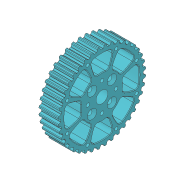
# Autodesk Inventor part: TIMING_BELT_P40
Saved by Autodesk Inventor 2019.4 (Build 234330000, 330)
## iProperties
Created: 2019-11-09
Part Number: TIMING_BELT_P40
Material: 一般
Document SubType Name: Modeling
Designer: y6tada
Density: 1 g/cm^3
Appearance: くすんだ青
Author: y6tada
Autodesk Inventor part; units mm, degrees
ref_plane "YZ Plane" through (0, 0, 0) normal (1, 0, 0) x (0, 1, 0)
ref_plane "XZ Plane" through (0, 0, 0) normal (0, 1, 0) x (-1, 0, 0)
ref_plane "XY Plane" through (0, 0, 0) normal (0, 0, 1) x (1, 0, 0)
sketch "スケッチ1" plane through (0, 0, 0) normal (1, 0, 0) x (0, 1, 0)
  arc A0 (0.9801, -18.6943) -> (0, -18.72) centre (0, 0) ccw construction
  line L0 (0, 0) -> (0, -15.5638) construction
  line L1 (0.975, -18.974) -> (-0.975, -18.974) construction
  arc A1 (0.9801, -18.6943) -> (0.4479, -17.6043) centre (-0.975, -18.974) ccw
  arc A2 (-0.4479, -17.6043) -> (0.4479, -17.6043) centre (0, 0) ccw
  arc A3 (-0.4479, -17.6043) -> (-0.9801, -18.6943) centre (0.975, -18.974) ccw
  circle A4 centre (0, 0) radius 14.32 construction
  line L2 (0, -18.72) -> (0.975, -18.72) construction
  circle A5 centre (0, 0) radius 19.1 construction
  line L3 (1.4688, -18.6623) -> (0, 0)
  line L4 (0, 0) -> (-1.4688, -18.6623)
  arc A6 (-1.4688, -18.6623) -> (-0.9801, -18.6943) centre (0, 0) ccw
  arc A7 (0.9801, -18.6943) -> (1.4688, -18.6623) centre (0, 0) ccw
  dimension "d2" = 1.95
  dimension "d3" = 1.975
  dimension "d4" = 1.11
  dimension "d8" = 0.254
  dimension "d10" = 37.44
  dimension "d11" = 38.2
  dimension "d12" = 9
  constraints: 14 point on circle, 10 end point, 8 centre point, 4 symmetric about line, 3 coincident, 1 concentric, 1 horizontal, 1 perpendicular, 1 point on line, 1 tangent, 1 vertical, 1 other
  measures "d2" distance of L1.start L1.end
  measures "d3" radius of A1
  measures "d4" radial gap between concentric circles of A0 A2
  measures "d8" distance between parallel lines of L1 L2
  measures "d10" diameter of A0
  measures "d11" diameter of A5
  measures "d12" angle of L4 L3
extrude "押し出し1" add sketch "スケッチ1" along normal blind 8.2
fillet "フィレット1" radius 0.15 2 edges at (4.1, 0.4479, -17.6043) (4.1, -0.4479, -17.6043)
fillet "フィレット2" radius 0.28 2 edges at (4.1, 0.9801, -18.6943) (4.1, -0.9801, -18.6943)
pattern_circular "円形状パターン1" count 40 over 360 about axis through (-10, 0, 0) along (1, 0, 0)
sketch "スケッチ9" plane through (0, 0, 0) normal (-1, 0, 0) x (0, 0, 1)
  circle A0 centre (0, 0) radius 14
  dimension "d79" = 28
  constraints: 1 centre point, 1 coincident
  measures "d79" diameter of A0
extrude "押し出し6" add sketch "スケッチ9" along normal blind 1
sketch "スケッチ3" plane through (-1, 0, 0) normal (-1, 0, 0) x (0, 0, 1)
  circle A0 centre (0, 0) radius 7.5
  dimension "d27" = 15
  constraints: 1 centre point, 1 coincident
  measures "d27" diameter of A0
extrude "押し出し2" add sketch "スケッチ3" along normal blind 1
sketch "スケッチ2" plane through (8.2, 0, 0) normal (1, 0, 0) x (0, 0, -1)
  point P0 (0, 0)
  point P1 (0, 0)
  constraints: 1 coincident
hole "穴1" at (8.2, 0, 0) direction (-1, 0, 0) diameter 5 end through all
sketch "スケッチ4" plane through (-2, 0, 0) normal (-1, 0, 0) x (0, 0, 1)
  circle A0 centre (0, 0) radius 6 construction
  line L0 (0, 0) -> (6, 0) construction
  point P0 (0, 6)
  point P1 (-6, 0)
  point P2 (0, -6)
  dimension "d30" = 12
  dimension "d33" = 360
  constraints: 2 end point, 1 coincident, 1 horizontal, 1 horizontal alignment, 7 other
hole "穴2" at (-2, 0, 6) at (-2, 6, 0) at (-2, 0, -6) at (-2, -6, 0) direction (1, 0, 0) diameter 1.5 end through all both
sketch "スケッチ5" plane through (8.2, 0, 0) normal (-1, 0, 0) x (0, 0, 1)
  circle A0 centre (0, 0) radius 6 construction
  line L0 (0, 0) -> (4.2426, 4.2426) construction
  line L1 (0, 0) -> (9.6781, 0) construction
  point P0 (-4.2426, 4.2426)
  point P1 (-4.2426, -4.2426)
  point P2 (4.2426, -4.2426)
  dimension "d43" = 12
  dimension "d42" = 45
  dimension "d46" = 360
  constraints: 4 end point, 2 coincident, 1 horizontal, 8 other
  measures "d42" angle of L1 L0
hole "穴3" at (8.2, 4.2426, 4.2426) at (8.2, 4.2426, -4.2426) at (8.2, -4.2426, -4.2426) at (8.2, -4.2426, 4.2426) direction (-1, 0, 0) diameter 2 end through all countersink diameter 4 countersink angle 90
sketch "スケッチ6" plane through (-1, 0, 0) normal (-1, 0, 0) x (0, 0, 1)
  circle A0 centre (0, 0) radius 8.4
  circle A1 centre (0, 0) radius 10.2
  dimension "d55" = 20.4
  dimension "d56" = 16.8
  constraints: 2 centre point, 2 coincident
  measures "d55" diameter of A1
  measures "d56" diameter of A0
extrude "押し出し3" cut sketch "スケッチ6" against normal blind 0.2
sketch "スケッチ7" plane through (-1, 0, 0) normal (-1, 0, 0) x (0, 0, 1)
  circle A0 centre (0, 0) radius 12 construction
  circle A1 centre (0, 0) radius 11.45
  circle A2 centre (0, 0) radius 12.55
  dimension "d59" = 24
  dimension "d60" = 0.55
  dimension "d61" = 0.55
  constraints: 3 centre point, 3 coincident
  measures "d59" diameter of A0
  measures "d60" radial gap between concentric circles of A0 A1
  measures "d61" radial gap between concentric circles of A2 A0
extrude "押し出し4" cut sketch "スケッチ7" against normal blind 0.5
sketch "スケッチ8" plane through (8.2, 0, 0) normal (1, 0, 0) x (0, 0, -1)
  circle A0 centre (0, 0) radius 9 construction
  circle A1 centre (0, 0) radius 16 construction
  line L0 (0, 0) -> (14.7821, 6.1229) construction
  line L1 (0, 0) -> (14.7821, -6.1229) construction
  line L2 (0, 0) -> (22.4689, 0) construction
  arc A2 (13.8872, 4.447) -> (9.7713, 3.1815) centre (18.5109, -17.9179) ccw
  arc A3 (8.8674, -1.5391) -> (8.8674, 1.5391) centre (0, 0) ccw
  arc A4 (15.6589, -3.2861) -> (15.6589, 3.2861) centre (0, 0) ccw
  arc A5 (9.7713, 3.1815) -> (8.8674, 1.5391) centre (10.3453, 1.7957) ccw
  arc A6 (15.6589, 3.2861) -> (13.8872, 4.447) centre (14.1909, 2.978) ccw
  arc A7 (9.7713, -3.1815) -> (13.8872, -4.447) centre (18.5109, 17.9179) ccw
  arc A8 (8.8674, -1.5391) -> (9.7713, -3.1815) centre (10.3453, -1.7957) ccw
  arc A9 (13.8872, -4.447) -> (15.6589, -3.2861) centre (14.1909, -2.978) ccw
  line L3 (0.6834, -0.5828) -> (15.4655, 5.5401) construction
  circle A10 centre (14.7821, 6.1229) radius 1.7 construction
  dimension "d64" = 18
  dimension "d65" = 32
  dimension "d66" = 45
  dimension "d67" = 1.5
  dimension "d69" = 1.6
  dimension "d83" = 3.4
  constraints: 18 point on circle, 11 centre point, 10 tangent, 8 end point, 5 coincident, 5 equal radius, 2 concentric, 2 symmetric about line, 1 horizontal, 1 parallel, 1 point on line, 1 other
  measures "d64" diameter of A0
  measures "d65" diameter of A1
  measures "d66" angle of L1 L0
  measures "d67" radius of A5
  measures "d69" diameter of L3 L0
  measures "d83" diameter of A10
extrude "押し出し5" cut sketch "スケッチ8" against normal blind 7
hole "穴4" at (8.2, 6.1229, -14.7821) direction (-1, 0, 0) diameter 1.4 end through all
chamfer "面取り1" distance 0.25 angle 45 8 edges at (8.2, 0, -16) (8.2, -4.2327, -15.013) (8.2, -3.9114, -11.7994) (8.2, -2.5189, -9.0312) (8.2, 0, -9) (8.2, 2.5189, -9.0312) (8.2, 3.9114, -11.7994) (8.2, 4.2327, -15.013)
pattern_circular "円形状パターン2" count 8 over 360 about axis through (-10, 0, 0) along (1, 0, 0) of "押し出し5", "面取り1", "穴4"
